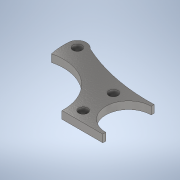
# Autodesk Inventor part: RCT-H111_upper_link_mount
Saved by Autodesk Inventor 2020 (Build 240168000, 168)
## iProperties
Created: 2019-12-05
Part Number: RCT-H111_upper_link_mount
Material: Generic
Document SubType Name: Modeling
Designer: maste
Density: 1 g/cm^3
Appearance: Galvanized
Author: maste
Autodesk Inventor part; units mm, degrees
ref_plane "YZ Plane" through (0, 0, 0) normal (1, 0, 0) x (0, 1, 0)
ref_plane "XZ Plane" through (0, 0, 0) normal (0, 1, 0) x (-1, 0, 0)
ref_plane "XY Plane" through (0, 0, 0) normal (0, 0, 1) x (1, 0, 0)
sketch "Sketch1" plane through (0, 0, 0) normal (0, 1, 0) x (-1, 0, 0)
  arc A0 (0, -7.5) -> (0, 7.5) centre (0, 0) ccw
  line L0 (0, 8.5) -> (17, 8.5)
  line L1 (17, 8.5) -> (17, -8.5) construction
  line L2 (17, -8.5) -> (0, -8.5) construction
  line L3 (0, 0) -> (10, 0) construction
  line L4 (10, 0) -> (10, -5) construction
  line L5 (10, -5) -> (0, -5) construction
  line L6 (0, -5) -> (0, 0) construction
  line L7 (0, 0) -> (10, 0) construction
  line L8 (10, 0) -> (10, 5) construction
  line L9 (10, 5) -> (0, 5) construction
  line L10 (0, 5) -> (0, 0) construction
  circle A1 centre (10, -5) radius 1.5
  circle A2 centre (10, 5) radius 1.5
  line L11 (0, -8.5) -> (0, -7.5)
  line L12 (0, 7.5) -> (0, 8.5)
  line L13 (11.5, -5) -> (32, -5) construction
  line L14 (32, -5) -> (32, 5) construction
  line L15 (32, 5) -> (11.5, 5) construction
  line L16 (11.5, 5) -> (11.5, -5) construction
  circle A3 centre (29, -12.06) radius 1.5
  arc A4 (26.6329, -13.9031) -> (32, -12.06) centre (29, -12.06) ccw
  arc A5 (32, -12.06) -> (17, 8.5) centre (12.4412, -10.5777) ccw
  arc A6 (26.6329, -13.9031) -> (0, -8.5) centre (1.8893, -67.5285) ccw
  dimension "d9" = 3
  dimension "d0" = 15
  dimension "d2" = 17
  dimension "d3" = 17
  dimension "d4" = 8.5
  dimension "d5" = 10
  dimension "d6" = 5
  dimension "d7" = 10
  dimension "d8" = 5
  dimension "d10" = 3
  dimension "d13" = 20.5
  dimension "d14" = 7.06
  dimension "d15" = 3
  dimension "d16" = 3
  dimension "d17" = 6
  constraints: 34 end point, 9 parallel, 8 point on circle, 6 centre point, 6 coincident, 4 horizontal, 4 perpendicular, 1 horizontal alignment, 2 other
  measures "d0" diameter of A0
  measures "d2" distance of L0.end L1.end
  measures "d3" distance of L1.end L2.end
  measures "d4" distance from line of point (0, 0) L2
  measures "d5" distance of L5.end L4.end
  measures "d6" distance of L3.end L4.end
  measures "d7" distance of L9.end L8.end
  measures "d8" distance of L7.end L8.end
  measures "d10" diameter of A2
  measures "d13" distance of L15.end L14.end
  measures "d14" vertical distance of point (29, -12.06) point (10, -5)
  measures "d15" distance from line of L14 point (29, -12.06)
  measures "d16" diameter of A3
  measures "d17" diameter of A4
extrude "Extrusion2" add sketch "Sketch1" along normal blind 2.5
sketch "Sketch2" plane through (0, 2.5, 0) normal (0, 1, 0) x (1, 0, 0)
  circle A0 centre (-28, -8) radius 14.4875
  point P0 (0, 0)
  dimension "d20" = 28
  dimension "d21" = 8
  constraints: 1 centre point
  measures "d20" horizontal distance of point (0, 0) A0.centre
  measures "d21" vertical distance of point (0, 0) A0.centre
extrude "Extrusion3" cut sketch "Sketch2" against normal through all
body "Solid2"
